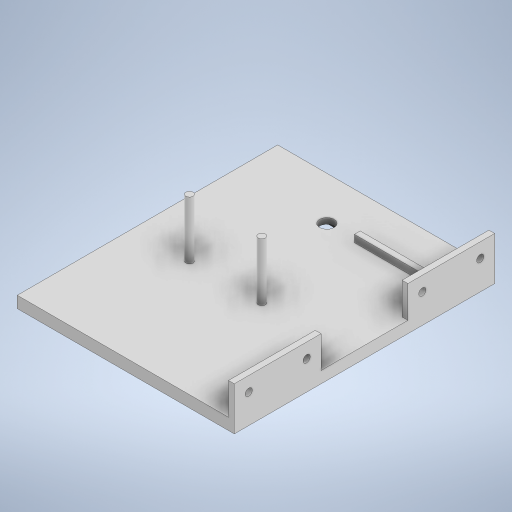
# Autodesk Inventor part: Стенка энкодера штурвала
Saved by Autodesk Inventor 2023 (Build 270158000, 158)
## iProperties
Created: 2022-05-17
Part Number: Стенка энкодера штурвала
Material: Типовые
Document SubType Name: Modeling
Designer: avkap
Density: 1 g/cm^3
Appearance: По умолчанию
Author: avkap
Autodesk Inventor part; units mm, degrees
ref_plane "YZ Plane" through (0, 0, 0) normal (1, 0, 0) x (0, 1, 0)
ref_plane "XZ Plane" through (0, 0, 0) normal (0, 1, 0) x (-1, 0, 0)
ref_plane "XY Plane" through (0, 0, 0) normal (0, 0, 1) x (1, 0, 0)
sketch "Эскиз1" plane through (0, 0, 0) normal (0, 1, 0) x (-1, 0, 0)
  line L0 (0, 0) -> (110, 0)
  line L1 (110, 0) -> (110, -60)
  line L2 (110, -60) -> (0, -60)
  line L3 (0, -60) -> (0, 0)
  line L4 (0, -60) -> (86, -60)
  line L5 (86, -60) -> (86, -30)
  line L6 (86, -30) -> (75, -30)
  line L7 (75, -30) -> (75, -38)
  line L8 (75, -30) -> (75, -22)
  line L9 (75, -22) -> (97, -22)
  line L10 (97, -22) -> (97, -38)
  line L11 (97, -38) -> (75, -38)
  line L12 (0, -60) -> (150, -60)
  line L13 (150, -60) -> (150, 120)
  line L14 (150, 120) -> (0, 120)
  line L15 (0, 120) -> (0, -60)
  dimension "d0" = 110
  dimension "d1" = 60
  dimension "d2" = 86
  dimension "d3" = 30
  dimension "d4" = 11
  dimension "d5" = 8
  dimension "d6" = 8
  dimension "d7" = 22
  dimension "d27" = 150
  dimension "d28" = 180
  constraints: 32 end point, 8 perpendicular, 4 parallel, 2 horizontal, 1 point on line, 1 vertical
  measures "d0" distance of L1.end L2.end
  measures "d1" distance of L0.end L1.end
  measures "d2" distance of L2.end L4.end
  measures "d3" distance of L4.end L5.end
  measures "d4" distance of L5.end L6.end
  measures "d5" distance of L6.end L7.end
  measures "d6" distance of L6.end L8.end
  measures "d7" distance of L8.end L9.end
  measures "d27" distance of L14.end L13.end
  measures "d28" distance of L13.end L12.end
extrude "Выдавливание1" add sketch "Эскиз1" along normal blind 4
sketch "Эскиз2" plane through (0, 4, 0) normal (0, 1, 0) x (1, 0, 0)
  line L0 (-110, 60) -> (-110, 0) projected
  line L1 (-110, 0) -> (0, 0)
  line L2 (0, 0) -> (0, 60)
  line L3 (0, 60) -> (-110, 60)
  line L4 (-110, 60) -> (-110, 0)
  circle A0 centre (-86, 30) radius 5
  line L5 (0, 60) -> (-150, 60) projected
  line L6 (0, 60) -> (-150, 60)
  line L7 (-150, 60) -> (-150, -120)
  line L8 (-150, -120) -> (0, -120)
  line L9 (0, -120) -> (0, 60)
  dimension "d10" = 10
  constraints: 16 end point, 4 parallel, 2 horizontal, 2 perpendicular, 1 centre point
  measures "d10" diameter of A0
extrude "Выдавливание2" add sketch "Эскиз2" along normal blind 4
sketch "Эскиз3" plane through (0, 8, 0) normal (0, 1, 0) x (1, 0, 0)
  line L0 (0, 0) -> (0, 60) projected
  line L1 (0, 30) -> (0, 28)
  line L2 (0, 28) -> (-65, 28)
  line L3 (-65, 28) -> (-65, 32)
  line L4 (-65, 32) -> (0, 32)
  line L5 (0, 32) -> (0, 28)
  point P0 (0, 32)
  dimension "d13" = 2
  dimension "d14" = 65
  dimension "d15" = 4
  constraints: 10 end point, 2 perpendicular, 2 point on line, 1 midpoint
  measures "d13" distance of L1.start L1.end
  measures "d14" distance of L1.end L2.end
  measures "d15" distance of L2.end L3.end
extrude "Выдавливание3" add sketch "Эскиз3" along normal blind 5
sketch "Эскиз5" plane through (0, 0, 120) normal (1, 0, 0) x (0, 0, -1)
  line L0 (180, 0) -> (120, 0)
  line L1 (120, 0) -> (120, 30)
  line L2 (120, 30) -> (180, 30)
  line L3 (180, 30) -> (180, 0)
  line L4 (180, 0) -> (0, 0) projected
  line L5 (0, 0) -> (60, 0)
  line L6 (60, 0) -> (60, 30)
  line L7 (60, 30) -> (0, 30)
  line L8 (0, 30) -> (0, 0)
  line L9 (60, 30) -> (60, 20)
  line L10 (60, 20) -> (50, 20)
  line L11 (0, 30) -> (0, 20)
  line L12 (0, 20) -> (10, 20)
  circle A0 centre (10, 20) radius 2.5
  circle A1 centre (50, 20) radius 2.5
  line L13 (120, 20) -> (130, 20)
  line L14 (180, 20) -> (170, 20)
  circle A2 centre (130, 20) radius 2.5
  circle A3 centre (170, 20) radius 2.5
  dimension "d29" = 60
  dimension "d30" = 30
  dimension "d31" = 60
  dimension "d32" = 30
  dimension "d33" = 10
  dimension "d34" = 10
  dimension "d35" = 10
  dimension "d36" = 10
  dimension "d37" = 5
  dimension "d38" = 5
  dimension "d39" = 10
  dimension "d40" = 10
  dimension "d41" = 5
  dimension "d42" = 5
  constraints: 28 end point, 7 point on line, 5 parallel, 4 centre point, 4 coincident, 3 perpendicular, 2 horizontal
  measures "d29" distance of L1.end L2.end
  measures "d30" distance of L0.end L1.end
  measures "d31" distance of L7.end L6.end
  measures "d32" distance of L6.end L5.end
  measures "d33" distance of L6.end L9.end
  measures "d34" distance of L9.end L10.end
  measures "d35" distance of L7.end L11.end
  measures "d36" distance of L11.end L12.end
  measures "d37" diameter of A0
  measures "d38" diameter of A1
  measures "d39" distance of L13.start L13.end
  measures "d40" distance of L14.start L14.end
  measures "d41" diameter of A2
  measures "d42" diameter of A3
extrude "Выдавливание5" add sketch "Эскиз5" against normal blind 4
sketch "Эскиз6" plane through (0, 8, 0) normal (0, 1, 0) x (1, 0, 0)
  circle A0 centre (-86, 30) radius 5 projected
  line L0 (-86, 30) -> (-86, -120)
  line L1 (-150, -120) -> (0, -120) projected
  line L2 (-86, -120) -> (-86, -100)
  circle A1 centre (-86, -100) radius 10
  circle A2 centre (-86, -100) radius 20
  circle A3 centre (-86, 30) radius 40
  line L3 (-105.7619, -103.0769) -> (-125.5238, 23.8462)
  line L4 (-66.2381, -103.0769) -> (-46.4762, 23.8462)
  line L5 (-86, -100) -> (-86, -40)
  line L6 (-86, -40) -> (-111, -40)
  line L7 (-86, -40) -> (-61, -40)
  circle A4 centre (-111, -40) radius 2.5
  circle A5 centre (-61, -40) radius 2.5
  point P0 (0, 0)
  dimension "d45" = 20
  dimension "d46" = 20
  dimension "d47" = 40
  dimension "d48" = 80
  dimension "d49" = 60
  dimension "d50" = 25
  dimension "d52" = 25
  dimension "d53" = 5
  dimension "d54" = 5
  constraints: 14 end point, 5 centre point, 5 coincident, 4 point on circle, 4 tangent, 3 point on line, 1 perpendicular, 1 vertical
  measures "d45" distance of L0.end L2.end
  measures "d46" diameter of A1
  measures "d47" diameter of A2
  measures "d48" diameter of A3
  measures "d49" distance of L5.start L5.end
  measures "d50" distance of L5.end L6.end
  measures "d52" distance of L5.end L7.end
  measures "d53" diameter of A4
  measures "d54" diameter of A5
extrude "Выдавливание6" add sketch "Эскиз6" along normal blind 40 contours A4 | A5
